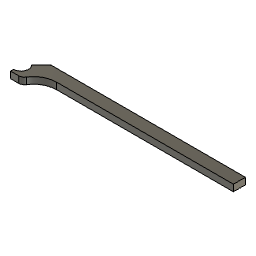
Finger1Section4P1V1 v2 (Autodesk Fusion 360 design; units mm, degrees)
Autodesk Fusion 360 part; units mm, degrees
sketch "Sketch1" plane through (0, 0, 0) normal (0, 0, 1) x (1, 0, 0)
  line L0 (3.507, 3) -> (2.507, 3)
  line L1 (4.507, 4) -> (5.507, 5)
  line L2 (5.507, 5) -> (20.507, 5)
  line L3 (2.2748, 1.7678) -> (3.507, 3)
  line L4 (0.507, -2.5) -> (0.507, -3.5)
  line L5 (0.507, -3.5) -> (3.2053, -3.5)
  line L6 (20.507, 5) -> (70.507, 5)
  line L7 (70.507, 3) -> (70.507, 1)
  line L8 (70.507, 5) -> (70.507, 4)
  line L9 (70.507, 1) -> (65.507, 1)
  line L10 (65.507, 1) -> (11.3814, 1)
  arc A0 (0.507, -2.5) -> (2.2748, 1.7678) centre (0.507, 0) ccw
  arc A1 (11.3814, 1) -> (4.895, -2.57) centre (11.3814, -6.6776) ccw
  arc A2 (3.2053, -3.5) -> (4.895, -2.57) centre (3.2053, -1.5) ccw
  line L11 (3.507, 3) -> (4.507, 4)
  line L12 (70.507, 3) -> (70.507, 4)
  dimension "d19" = 50
  dimension "d20" = 2
  dimension "d24" = 5
  dimension "d29" = 5
  dimension "d30" = 2
  constraint horizontal L0
  constraint perpendicular L4 L5
  constraint perpendicular L5 L7
  constraint perpendicular L7 L9
  constraint tangent L10 A1
  constraint tangent L5 A2
  constraint tangent A1 A2
  constraint parallel L1 L11
  measures "d19" distance of L2.end L6.end
  measures "d20" distance of L7.start L7.end
  measures "d24" distance of L7.end L9.end
  measures "d29" diameter of A0
  measures "d30" radius of A2
extrude "Extrude5" add sketch "Sketch1" along normal blind 2.2
